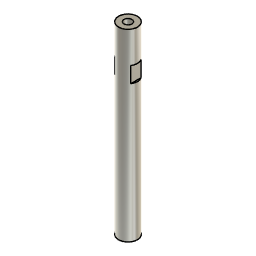
MIDDLE_ROD (Autodesk Fusion 360 design; units mm, degrees)
Autodesk Fusion 360 part; units mm, degrees
sketch "Esquisse1" plane through (0, 0, 0) normal (0, 0, 1) x (1, 0, 0)
  circle A0 centre (0, 0) radius 6
  dimension "d1" = 12
  constraint coincident A0.centre origin
  measures "d1" diameter of A0
extrude "Extrusion1" add sketch "Esquisse1" along normal blind 117
sketch "Esquisse2" plane through (0, 0, 117) normal (0, 0, 1) x (-1, 0, 0)
  circle A0 centre (0, 0) radius 6
  circle A1 centre (0, 0) radius 2.5
  dimension "d5" = 5
  constraint coincident A0.centre A1.centre
  measures "d5" diameter of A1
extrude "Extrusion2" cut sketch "Esquisse2" against normal blind 12 contours A1
sketch "Esquisse3" plane through (0, 0, 0) normal (0, 0, -1) x (1, 0, 0)
  circle A0 centre (0, 0) radius 6
  circle A1 centre (0, 0) radius 2.5
  dimension "d8" = 5
  constraint concentric A0 A1
  measures "d8" diameter of A1
extrude "Extrusion3" cut sketch "Esquisse3" against normal blind 12 contours A1
sketch "Esquisse4" plane through (0, 0, 117) normal (0, 0, 1) x (-1, 0, 0)
  circle A0 centre (0, 0) radius 2.5
  circle A1 centre (0, 0) radius 6
  line L0 (5, 8) -> (-5, 8)
  line L1 (-5, 8) -> (-5, -7.4606)
  line L2 (-5, -7.4606) -> (5, -7.4606)
  line L3 (5, -7.4606) -> (5, 8)
  dimension "d11" = 5
  dimension "d12" = 10
  constraint horizontal L0
  constraint vertical L1
  constraint horizontal L2
  constraint vertical L3
  measures "d11" distance of A0.centre L1
  measures "d12" distance of L1.end L2.end
extrude "Extrusion4" cut sketch "Esquisse4" against normal blind 10 from surface at -20 contours A1 L3 | A1 L1
